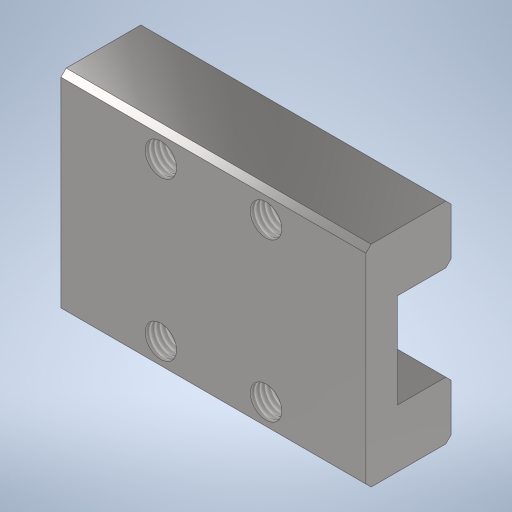
# Autodesk Inventor part: slider
Saved by Autodesk Inventor 2024 (Build 280153000, 153)
## iProperties
Created: 2025-06-01
Part Number: slider
Material: ステンレス鋼
Document SubType Name: Modeling
Designer: 1412z
Density: 8 g/cm^3
Appearance: 半つや出し
Author: 1412z
Autodesk Inventor part; units mm, degrees
ref_plane "YZ Plane" through (0, 0, 0) normal (1, 0, 0) x (0, 1, 0)
ref_plane "XZ Plane" through (0, 0, 0) normal (0, 1, 0) x (-1, 0, 0)
ref_plane "XY Plane" through (0, 0, 0) normal (0, 0, 1) x (1, 0, 0)
sketch "スケッチ1" plane through (0, 0, 0) normal (0, 0, 1) x (1, 0, 0)
  line L0 (14.5, 10) -> (-14.5, 10)
  line L1 (-14.5, 10) -> (-14.5, -10)
  line L2 (-14.5, -10) -> (14.5, -10)
  line L3 (14.5, -10) -> (14.5, 10)
  line L4 (14.5, 10) -> (-14.5, -10) construction
  line L5 (-14.5, 10) -> (14.5, -10) construction
  point P0 (0, 0)
  dimension "d0" = 29
  dimension "d1" = 20
  constraints: 12 end point, 2 midpoint, 2 parallel, 1 horizontal, 1 perpendicular
  measures "d0" distance of L2.end L1.end
  measures "d1" distance of L1.end L0.end
extrude "押し出し1" add sketch "スケッチ1" along normal blind 8.1
sketch "スケッチ2" plane through (0, 0, 8.1) normal (0, 0, 1) x (1, 0, 0)
  circle A0 centre (-5, 7.5) radius 1.5
  circle A1 centre (5, 7.5) radius 1.5
  circle A2 centre (5, -7.5) radius 1.5
  circle A3 centre (-5, -7.5) radius 1.5
  point P0 (0, 0)
  dimension "d4" = 3
  dimension "d5" = 3
  dimension "d6" = 3
  dimension "d7" = 3
  constraints: 4 centre point
  measures "d4" diameter of A0
  measures "d5" diameter of A1
  measures "d6" diameter of A2
  measures "d7" diameter of A3
extrude "押し出し2" cut sketch "スケッチ2" against normal blind 4
thread "ねじ1" size "M3x0.5" class "6H" standard "ANSI Metric M Profile" full length
thread "ねじ2" size "M3x0.5" class "6H" standard "ANSI Metric M Profile" full length
thread "ねじ3" size "M3x0.5" class "6H" standard "ANSI Metric M Profile" full length
thread "ねじ4" size "M3x0.5" class "6H" standard "ANSI Metric M Profile" full length
sketch "スケッチ3" plane through (0, 0, 0) normal (0, 0, -1) x (-1, 0, 0)
  line L0 (-14.5, -10) -> (-14.5, 10) projected
  line L1 (14.5, -4.5) -> (-14.5, -4.5)
  line L2 (-14.5, -4.5) -> (-14.5, 4.5)
  line L3 (-14.5, 4.5) -> (14.5, 4.5)
  line L4 (14.5, 4.5) -> (14.5, -4.5)
  line L5 (14.5, -4.5) -> (-14.5, 4.5) construction
  line L6 (-14.5, -4.5) -> (14.5, 4.5) construction
  point P0 (0, 0)
  dimension "d18" = 9
  constraints: 12 end point, 2 midpoint, 2 parallel, 1 horizontal, 1 perpendicular, 1 point on line
  measures "d18" distance of L1.end L2.end
extrude "押し出し3" cut sketch "スケッチ3" against normal blind 5.1
chamfer "面取り1" distance 0.5 angle 45 6 edges at (0, 10, 8.1) (0, -10, 8.1) (0, -10, 0) (0, 10, 0) (0, -4.5, 0) (0, 4.5, 0)
